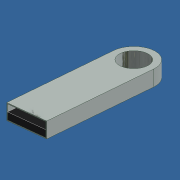
# Autodesk Inventor part: Metal USB stick with hole
Saved by Autodesk Inventor 2021 (Build 250183000, 183)
## iProperties
Manager: -
Created: 2022-08-08
Part Number: Metal USB stick with hole
Material: Acero
Document SubType Name: Modeling
Designer: Usuario
Density: 8 g/cm^3
Appearance: Cinc
Author: Usuario
Revision Number: 01
Autodesk Inventor part; units mm, degrees
ref_plane "YZ Plane" through (0, 0, 0) normal (1, 0, 0) x (0, 1, 0)
ref_plane "XZ Plane" through (0, 0, 0) normal (0, 1, 0) x (-1, 0, 0)
ref_plane "XY Plane" through (0, 0, 0) normal (0, 0, 1) x (1, 0, 0)
sketch "Boceto1" plane through (0, 0, 0) normal (0, 0, 1) x (1, 0, 0)
  line L0 (6.125, 0) -> (-6.125, 0)
  line L1 (-6.125, 0) -> (-6.125, 33.675)
  circle A0 centre (0, 33.675) radius 4.15
  arc A1 (6.125, 33.675) -> (-6.125, 33.675) centre (0, 33.675) ccw
  line L2 (6.125, 0) -> (6.125, 33.675)
  point P0 (0, 0)
  point P1 (0, 0)
  dimension "d44" = 39.8
  dimension "d45" = 12.25
  dimension "d46" = 8.3
  constraints: 6 end point, 2 centre point, 2 coincident, 2 point on circle, 2 tangent, 1 horizontal, 1 midpoint, 1 perpendicular, 1 vertical alignment
  measures "d45" distance between parallel lines of L2 L1
  measures "d46" diameter of A0
extrude "Extrusión4" add sketch "Boceto1" along normal mid plane 4.5
sketch "Boceto7" plane through (-6.125, 0, 2.25) normal (0, -1, 0) x (1, 0, 0)
  line L0 (12, -4.25) -> (0.25, -4.25)
  line L1 (0.25, -4.25) -> (0.25, -0.25)
  line L2 (0.25, -0.25) -> (12, -0.25)
  line L3 (12, -0.25) -> (12, -4.25)
  line L4 (12, -4.25) -> (0.25, -0.25) construction
  line L5 (0.25, -4.25) -> (12, -0.25) construction
  line L6 (0, 0) -> (12.25, 0) projected
  line L7 (0, -4.5) -> (0, 0) projected
  point P0 (6.125, -2.25)
  dimension "d49" = 0.25
  dimension "d50" = 0.25
  constraints: 12 end point, 2 midpoint, 2 parallel, 1 horizontal, 1 perpendicular
  measures "d49" distance between parallel lines of L2 L6
  measures "d50" distance between parallel lines of L7 L1
extrude "Extrusión5" cut sketch "Boceto7" against normal blind 10.5
sketch "Boceto8" plane through (-6.125, 0, 2.25) normal (0, -1, 0) x (1, 0, 0)
  line L0 (0.25, -4.25) -> (0.25, -0.25) construction
  line L1 (0.25, -0.25) -> (12, -0.25) construction
  line L2 (12, -0.25) -> (12, -4.25) construction
  line L3 (12, -4.25) -> (0.25, -4.25) construction
  line L4 (12.25, -4.5) -> (12.25, 0) construction
  line L5 (0, 0) -> (12.25, 0) construction
  line L6 (0, -4.5) -> (0, 0) construction
  line L7 (12.25, -4.5) -> (0, -4.5) construction
  line L8 (12, -4.25) -> (0.25, -4.25) projected
  line L9 (12, -0.25) -> (12, -4.25) projected
  line L10 (0.25, -4.25) -> (12, -4.25)
  line L11 (12, -4.25) -> (12, -2.25)
  line L12 (12, -2.25) -> (0.25, -2.25)
  line L13 (0.25, -2.25) -> (0.25, -4.25)
  point P0 (6.125, -2.25)
  constraints: 8 end point, 2 midpoint, 2 parallel, 1 horizontal, 1 perpendicular
extrude "Extrusión6" add sketch "Boceto8" against normal up to surface (10.5 mm away) separate body
equation "\"d50\" = d49"
